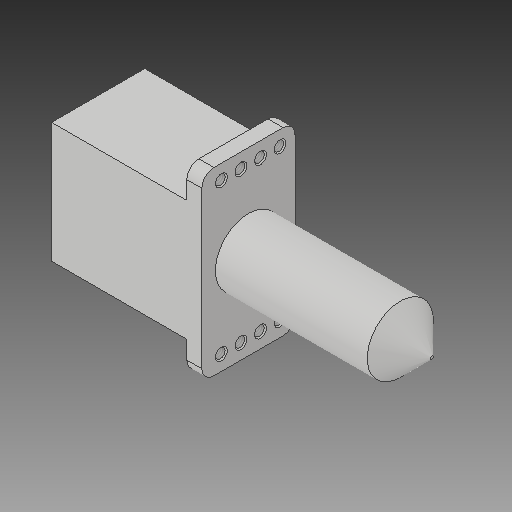
# Autodesk Inventor part: GT9S Extruder
Saved by Autodesk Inventor 2019 (Build 230136000, 136)
## iProperties
Created: 2018-10-20
Part Number: GT9S Extruder
Material: Generic
Document SubType Name: Modeling
Designer: LillaHunden
Density: 1 g/cm^3
Appearance: Default
Mass: 85.6152 g
Surface Area: 152.974 cm^2
Volume: 85.6152 cm^3
Author: LillaHunden
Autodesk Inventor part; units mm, degrees
ref_plane "YZ Plane" through (0, 0, 0) normal (1, 0, 0) x (0, 1, 0)
ref_plane "XZ Plane" through (0, 0, 0) normal (0, 1, 0) x (-1, 0, 0)
ref_plane "XY Plane" through (0, 0, 0) normal (0, 0, 1) x (1, 0, 0)
sketch "Sketch1" plane through (0, 0, 0) normal (1, 0, 0) x (0, 1, 0)
  line L0 (-30, -15.5) -> (30, -15.5)
  line L1 (30, -15.5) -> (30, 15.5)
  line L2 (30, 15.5) -> (-30, 15.5)
  line L3 (-30, 15.5) -> (-30, -15.5)
  line L4 (-30, -15.5) -> (30, 15.5) construction
  line L5 (30, -15.5) -> (-30, 15.5) construction
  point P0 (0, 0)
  dimension "d0" = 60
  dimension "d1" = 31
  constraints: 12 end point, 2 midpoint, 2 parallel, 1 horizontal, 1 perpendicular
  measures "d0" distance of L1.end L2.end
  measures "d1" distance of L0.end L1.end
extrude "Extrusion1" add sketch "Sketch1" along normal blind 5
fillet "Fillet1" radius 4 4 edges at (2.5, 30, 15.5) (2.5, 30, -15.5) (2.5, -30, -15.5) (2.5, -30, 15.5)
sketch "Sketch2" plane through (5, 0, 0) normal (1, 0, 0) x (0, 0, -1)
  line L0 (-15.5, 26) -> (-15.5, -26) projected
  line L1 (11.5, 30) -> (-11.5, 30) projected
  point P0 (0, 0)
  point P1 (-9, 25.0416)
  point P2 (-9, -24.9584)
  point P3 (-2.5, 25.0416)
  point P4 (-2.5, -24.9584)
  point P5 (4, 25.0416)
  point P6 (4, -24.9584)
  point P7 (10.5, 25.0416)
  point P8 (10.5, -24.9584)
  dimension "d5" = 6.5
  dimension "d8" = 50
  dimension "d11" = 6.5
  constraints: 1 horizontal, 1 vertical, 7 other
  measures "d5" distance from line of L0 point (-9, 25.042)
  measures "d8" distance of point (-9, 25.042) point (-9, -24.958)
  measures "d11" distance of point (-9, 25.042) point (-2.5, 25.042)
hole "Hole1" at (5, 25.0416, 9) at (5, -24.9584, 9) at (5, 25.0416, 2.5) at (5, -24.9584, 2.5) at (5, 25.0416, -4) at (5, -24.9584, -4) at (5, 25.0416, -10.5) at (5, -24.9584, -10.5) direction (-1, 0, 0) diameter 3.242 depth 11.8 tip angle 118 countersink diameter 4 countersink angle 90 thread size "M4x0.7" class "6H" standard "ISO Metric profile"
sketch "Sketch3" plane through (5, 0, 0) normal (1, 0, 0) x (0, 0, -1)
  circle A0 centre (0, 0) radius 4
  dimension "d21" = 8
  constraints: 1 centre point, 1 coincident
  measures "d21" diameter of A0
extrude "Extrusion2" cut sketch "Sketch3" against normal blind 5
sketch "Sketch4" plane through (0, -26, 15.5) normal (0, 0, 1) x (1, 0, 0)
  line L0 (0, 0) -> (0, 52) projected
  line L1 (0, 6) -> (-45, 6)
  line L2 (-45, 6) -> (-45, 46)
  line L3 (-45, 46) -> (0, 46)
  line L4 (0, 46) -> (0, 6)
  line L5 (5, 52) -> (5, 0) projected
  line L6 (0, 26) -> (-7.0205, 26) construction
  dimension "d24" = 50
  dimension "d25" = 40
  constraints: 10 end point, 2 horizontal, 2 parallel, 1 perpendicular, 1 point on line, 1 other
  measures "d24" distance between parallel lines of L2 L5
  measures "d25" distance between parallel lines of L3 L1
extrude "Extrusion3" add sketch "Sketch4" against normal up to surface (31 mm away)
sketch "Sketch5" plane through (-45, -20, 15.5) normal (-1, 0, 0) x (0, 0, 1)
  circle A0 centre (-15.5, 20) radius 5.4211
  constraints: 1 centre point, 1 coincident
extrude "Extrusion4" add sketch "Sketch5" along normal blind 6
sketch "Sketch6" plane through (5, 0, 0) normal (1, 0, 0) x (0, 0, -1)
  circle A0 centre (0, 0) radius 11.0071
  constraints: 1 centre point, 1 coincident
extrude "Extrusion5" add sketch "Sketch6" along normal blind 61
chamfer "Chamfer1" distance 10.5 angle 45 1 edges at (66, 0, 11.0071)
body "Solid1"
